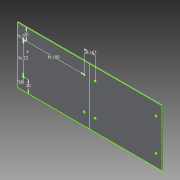
# Autodesk Inventor part: AlsoLemezVizhutes
Saved by Autodesk Inventor 2015 (Build 190159000, 159)
## iProperties
Created: 2014-10-31
Part Number: AlsoLemezVizhutes
Material: Generic
Document SubType Name: Modeling
Designer: laca
Density: 1 g/cm^3
Appearance: Default
d0: 108.000 mm
d1: 60.000 mm
JukaKoztiTavolsagHoszusag: 100.000 mm
JukakKoztiTavolsagSzeleseg: 53.000 mm
d4: 3.500 mm
d5: 4.000 mm
JukakANyakon: 3.000 mm
d7: 3.000 mm
d8: 3.000 mm
d9: 3.000 mm
d10: 1.500 mm
d11: 0.00 deg
d12: 1.500 mm
d13: 0.00 deg
d17: 8.000 mm
d18: 0.00 deg
d19: 10.000 mm
d20: 25.000 mm
d21: 1.100 mm
d22: 1.100 mm
d23: 0.200 mm
d26: 6.000 ul
d28: 2.450 mm
d29: 42.000 mm
d30: 8.000 mm
d31: 1.500 mm
d32: 1.000 mm
d33: 1.500 mm
d34: 1.000 mm
d35: 1.500 mm
d36: 1.000 mm
d37: 0.667 mm
d38: 0.667 mm
d40: 4.000 mm
d41: 0.00 deg
d42: 10.000 mm
d43: 5.000 mm
d44: 2.083 mm
d45: 1.500 mm
d47: 9.000 mm
d48: 0.00 deg
d49: 1.500 mm
d50: 6.500 mm
d51: 0.00 deg
d52: 3.500 mm
d54: 25.00 deg
d55: 4.000 ul
d57: 12.000 mm
TranzisztoJukAtmero: 4.000 mm
d59: 5.000 mm
d60: 3.000 mm
d62: 0.00 deg
d63: 12.000 mm
d64: 52.000 mm
d65: 4.000 mm
d66: 8.000 mm
d69: 6.000 mm
d70: 0.00 deg
d71: 1.000 mm
d72: 5.000 mm
d73: 0.00 deg
d74: 7.000 ul
d76: 8.497 mm
d77: 10.000 mm
d78: 10.000 mm
d79: 0.000 mm
d80: 11.000 mm
d81: 30.000 mm
d82: 20.000 mm
d83: 0.00 deg
d84: 1.000 mm
d2: 3.000 mm
d3: 2.000 ul
d14: 53.000 mm
d15: 2.000 ul
d24: 100.000 mm
d39: 20.000 mm
d46: 20.000 mm
d53: 10.000 mm
d61: 1.500 mm
d67: 0.00 deg
d68: 18.167 mm
Author: laca
Autodesk Inventor part; units mm, degrees
ref_plane "YZ Plane" through (0, 0, 0) normal (1, 0, 0) x (0, 1, 0)
ref_plane "XZ Plane" through (0, 0, 0) normal (0, 1, 0) x (-1, 0, 0)
ref_plane "XY Plane" through (0, 0, 0) normal (0, 0, 1) x (1, 0, 0)
sketch "Sketch1" plane through (0, 0, 0) normal (0, 1, 0) x (-1, 0, 0)
  circle A0 centre (7.2361, 13.6424) radius 1.5
  line L0 (0, 1.6974) -> (0, -1.2933)
  line L1 (1.3539, 0) -> (-1.1645, 0)
  circle A1 centre (7.2361, -39.3576) radius 1.5
  circle A2 centre (-92.7639, 13.6424) radius 1.5
  circle A3 centre (-92.7639, -39.3576) radius 1.5
  line L2 (17.2361, 33.6424) -> (-101.8474, 33.6424)
  line L3 (-101.8474, 33.6424) -> (-101.8474, -59.3576)
  line L4 (-101.8474, -59.3576) -> (17.2361, -59.3576)
  line L5 (17.2361, -59.3576) -> (17.2361, 33.6424)
  circle A4 centre (-210.9309, 13.6424) radius 1.5
  circle A5 centre (-210.9309, -39.3576) radius 1.5
  circle A6 centre (-110.9309, 13.6424) radius 1.5
  circle A7 centre (-110.9309, -39.3576) radius 1.5
  line L6 (-220.9309, 33.6424) -> (-101.8474, 33.6424)
  line L7 (-101.8474, -59.3576) -> (-220.9309, -59.3576)
  line L8 (-220.9309, -59.3576) -> (-220.9309, 33.6424)
  point P0 (0, 0)
  dimension "d2" = 3
  dimension "d14" = 53
  dimension "d24" = 100
  dimension "d39" = 20
  dimension "d46" = 20
  dimension "d53" = 10
  dimension "d68" = 18.167
  constraints: 18 end point, 8 centre point, 6 symmetric about line, 3 horizontal, 2 parallel, 2 vertical, 1 perpendicular, 10 other
  measures "d2" diameter of A0
  measures "d14" distance of A0.centre A1.centre
  measures "d24" distance of A0.centre A2.centre
  measures "d39" distance from line of A0.centre L2
  measures "d46" distance from line of L4 A1.centre
  measures "d53" distance from line of L5 A1.centre
  measures "d68" distance of A6.centre A2.centre
extrude "Extrusion1" add sketch "Sketch1" along normal blind 1.5
equation "\"d2\" = JukakANyakon"
equation "\"d14\" = JukakKoztiTavolsagSzeleseg"
equation "\"d24\" = JukaKoztiTavolsagHoszusag"
equation "\"JukakANyakon\" = 3"
equation "\"JukakKoztiTavolsagSzeleseg\" = 53"
equation "\"JukaKoztiTavolsagHoszusag\" = 100"
body "Solid1"
